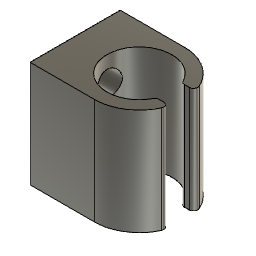
Mountable Linear Bearing Holder (Autodesk Fusion 360 design; units mm, degrees)
Autodesk Fusion 360 part; units mm, degrees
sketch "Sketch1" plane through (0, 0, 0) normal (0, 0, 1) x (1, 0, 0)
  line L0 (17.5, 3) -> (-7.01, 3)
  line L1 (17.5, -3) -> (17.5, 3)
  arc A0 (7.01, 3) -> (7.01, -3) centre (0, 0) ccw
  arc A1 (10.1927, 3) -> (10.1927, -3) centre (0, 0) ccw
  line L2 (-7.01, -3) -> (17.5, -3)
  dimension "d1" = 15.25
  constraint horizontal L0
  constraint coincident L0 A0.start
  constraint coincident L0 A1.start
  constraint coincident A0 L0.end
  constraint coincident A0 L2.start
  measures "d1" diameter of A0
extrude "Extrude1" add sketch "Sketch1" along normal blind 25 contours L0 A0 A1 L2 makes body 1
sketch "Sketch3" plane through (0, 0, 0) normal (0, 0, 1) x (1, 0, 0)
  arc A0 (7.01, 3) -> (7.01, -3) centre (0, 0) ccw construction
  line L0 (0, -10.625) -> (-15.125, -10.625)
  line L1 (-15.125, -10.625) -> (-15.125, 10.625)
  line L2 (-15.125, 10.625) -> (0, 10.625)
  arc A1 (10.1927, 3) -> (10.1927, -3) centre (0, 0) ccw
  line L3 (0, 10.625) -> (0, 7.625)
  line L4 (0, -7.625) -> (0, -10.625)
  constraint perpendicular L0 L3
  constraint parallel L1 L3
  constraint parallel L0 L2
  constraint coincident L0.start A1
  constraint vertical L3
  constraint coincident L2.end A1
  constraint coincident A0 L3.end
  constraint coincident A0 L4.start
  constraint collinear L3 L4
extrude "Extrude2" add sketch "Sketch3" along normal blind 25 bodies 1
ref_plane "WorkPlane1" through (-12.125, 0, 12.5) normal (-1, 0, 0) x (0, -1, 0)
sketch "Sketch4" plane through (-15.125, 0, 0) normal (-1, 0, 0) x (0, -1, 0)
  line L0 (-10.625, 0) -> (10.625, 0)
  line L1 (10.625, 0) -> (10.625, 25)
  line L2 (10.625, 25) -> (-10.625, 25)
  line L3 (-10.625, 25) -> (-10.625, 0)
  line L4 (0, 25) -> (0, 19) construction
  line L5 (0, 0) -> (0, 6) construction
  dimension "d11" = 6
  dimension "d12" = 6
  constraint midpoint L2 L4.start
  constraint perpendicular L2 L4
  constraint coincident L5.start origin
  constraint perpendicular L0 L5
  measures "d11" distance of L4.start L4.end
  measures "d12" distance of L5.start L5.end
hole "Hole1" at (-15.125, 0, 19) direction (1, 0, 0) diameter 3 end through all bodies 1
hole "Hole2" at (-15.125, 0, 6) direction (1, 0, 0) diameter 3 depth 24.216 tip angle 180 bodies 1
ref_plane "WorkPlane2" through (-5.125, 0, 12.5) normal (-1, 0, 0) x (0, -1, 0)
sketch "Sketch5" plane through (-5.125, 0, 12.5) normal (-1, 0, 0) x (0, 1, 0)
  line L0 (7.625, -12.5) -> (-7.625, -12.5) construction
  line L1 (0, -12.5) -> (0, -6.5) construction
  line L2 (-10.625, 12.5) -> (10.625, 12.5) construction
  line L3 (0, 12.5) -> (0, 6.5) construction
  point P0 (0, -12.5)
  point P1 (0, 12.5)
  dimension "d20" = 6
  dimension "d21" = 6
  constraint coincident P0 L1.start
  constraint perpendicular L0 L1
  constraint coincident P1 L3.start
  constraint perpendicular L2 L3
  measures "d20" distance of P0 L1.end
  measures "d21" distance of P1 L3.end
hole "Hole3" at (-5.125, 0, 19) direction (-1, 0, 0) diameter 6 end up to surface (7 mm away) bodies 1
hole "Hole4" at (-5.125, 0, 6) direction (-1, 0, 0) diameter 6 end up to surface (7 mm away) bodies 1
fillet "Fillet1" radius 1 4 edges at (10.1927, -3, 12.5) (7.01, -3, 12.5) (10.1927, 3, 12.5) (7.01, 3, 12.5) on bodies 1
copy_body "Body->Comp1" bodies 1 removing the originals makes body 2 in component "Mountable Linear Bearing Holder"
component "Mountable Linear Bearing Holder" placed x (1, 0, 0) y (0, 1, 0) z (0, 0, 1) at (0, 0, 0)
